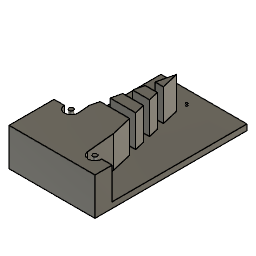
finger_v4_cast_p1 (Autodesk Fusion 360 design; units mm, degrees)
Autodesk Fusion 360 part; units mm, degrees
note: some values were not read from the file. Set by a fixed rule: which sketch regions a step uses.
sketch "Sketch1" plane through (0, 0, 0) normal (0, 0, 1) x (1, 0, 0)
  circle A0 centre (11, 11) radius 1.925
  circle A1 centre (11, 11) radius 3.8
  line L0 (11, 11) -> (56.3, 11) construction
  circle A2 centre (56.3, 11) radius 1.925
  circle A3 centre (56.3, 11) radius 3.8
  line L1 (11, 11) -> (11, 61.7133) construction
  line L2 (11, 11) -> (-8.4114, 83.4444) construction
  line L3 (-8.4114, 83.4444) -> (56.3, 11) construction
  line L4 (11, 11) -> (7.556, 12.6059) construction
  line L5 (11, 11) -> (13.1796, 14.1128) construction
  line L6 (10.0165, 14.6705) -> (8.9812, 18.5342) construction
  line L7 (5.9073, 19.5741) -> (5.1309, 22.4719)
  line L8 (6.3316, 20.3089) -> (5.8657, 22.0476)
  line L9 (5.8657, 22.0476) -> (8.1839, 22.6688)
  line L10 (5.1309, 22.4719) -> (7.4491, 23.093)
  line L11 (8.1839, 22.6688) -> (7.4075, 25.5665)
  line L12 (7.4491, 23.093) -> (6.9832, 24.8317)
  line L13 (6.9832, 24.8317) -> (4.665, 24.2105)
  line L14 (7.4075, 25.5665) -> (5.0893, 24.9454)
  line L15 (4.665, 24.2105) -> (3.8885, 27.1083)
  line L16 (5.0893, 24.9454) -> (4.6234, 26.684)
  line L17 (3.8885, 27.1083) -> (6.2068, 27.7295)
  line L18 (4.6234, 26.684) -> (6.9416, 27.3052)
  line L19 (6.2068, 27.7295) -> (5.7409, 29.4681)
  line L20 (6.9416, 27.3052) -> (6.1652, 30.203)
  line L21 (5.7409, 29.4681) -> (3.4227, 28.847)
  line L22 (6.1652, 30.203) -> (3.8469, 29.5818)
  line L23 (3.4227, 28.847) -> (2.6462, 31.7447)
  line L24 (3.8469, 29.5818) -> (3.3811, 31.3205)
  line L25 (2.6462, 31.7447) -> (4.9644, 32.3659)
  line L26 (3.3811, 31.3205) -> (5.6993, 31.9416)
  line L27 (4.9644, 32.3659) -> (4.4986, 34.1046)
  line L28 (5.6993, 31.9416) -> (4.9228, 34.8394)
  line L29 (4.4986, 34.1046) -> (2.1803, 33.4834)
  line L30 (4.9228, 34.8394) -> (2.6046, 34.2183)
  line L31 (2.1803, 33.4834) -> (1.4039, 36.3812)
  line L32 (2.6046, 34.2183) -> (2.1387, 35.9569)
  line L33 (1.4039, 36.3812) -> (3.7221, 37.0024)
  line L34 (2.1387, 35.9569) -> (4.457, 36.5781)
  line L35 (3.7221, 37.0024) -> (3.2562, 38.741)
  line L36 (4.457, 36.5781) -> (3.6805, 39.4759)
  line L37 (3.2562, 38.741) -> (0.938, 38.1199)
  line L38 (3.6805, 39.4759) -> (1.3623, 38.8547)
  line L39 (0.938, 38.1199) -> (0.1616, 41.0176)
  line L40 (1.3623, 38.8547) -> (0.8964, 40.5934)
  line L41 (0.1616, 41.0176) -> (2.4798, 41.6388)
  line L42 (0.8964, 40.5934) -> (3.2146, 41.2145)
  line L43 (2.4798, 41.6388) -> (2.0139, 43.3775)
  line L44 (3.2146, 41.2145) -> (2.4382, 44.1123)
  line L45 (2.0139, 43.3775) -> (-0.3043, 42.7563)
  line L46 (2.4382, 44.1123) -> (0.1199, 43.4911)
  line L47 (-0.3043, 42.7563) -> (-1.0808, 45.6541)
  line L48 (0.1199, 43.4911) -> (-0.3459, 45.2298)
  line L49 (-1.0808, 45.6541) -> (1.2374, 46.2752)
  line L50 (-0.3459, 45.2298) -> (1.9723, 45.851)
  line L51 (1.2374, 46.2752) -> (0.7716, 48.0139)
  line L52 (1.9723, 45.851) -> (1.1958, 48.7488)
  line L53 (0.7716, 48.0139) -> (-1.5467, 47.3927)
  line L54 (1.1958, 48.7488) -> (-1.1224, 48.1276)
  line L55 (-1.5467, 47.3927) -> (-2.3231, 50.2905)
  line L56 (-1.1224, 48.1276) -> (-1.5883, 49.8663)
  line L57 (-2.3231, 50.2905) -> (-0.0049, 50.9117)
  line L58 (-1.5883, 49.8663) -> (0.73, 50.4874)
  line L59 (-0.0049, 50.9117) -> (-0.4708, 52.6504)
  line L60 (0.73, 50.4874) -> (-0.0465, 53.3852)
  line L61 (-0.4708, 52.6504) -> (-2.789, 52.0292)
  line L62 (-0.0465, 53.3852) -> (-2.3647, 52.764)
  line L63 (-2.789, 52.0292) -> (-3.5654, 54.927)
  line L64 (-2.3647, 52.764) -> (-2.8306, 54.5027)
  line L65 (-3.5654, 54.927) -> (-1.2472, 55.5481)
  line L66 (-2.8306, 54.5027) -> (-0.5124, 55.1239)
  line L67 (-1.2472, 55.5481) -> (-1.7131, 57.2868)
  line L68 (-0.5124, 55.1239) -> (-1.2888, 58.0216)
  line L69 (-1.7131, 57.2868) -> (-4.0313, 56.6656)
  line L70 (-1.2888, 58.0216) -> (-3.607, 57.4005)
  line L71 (-4.0313, 56.6656) -> (-4.8078, 59.5634)
  line L72 (-3.607, 57.4005) -> (-4.0729, 59.1391)
  line L73 (-4.8078, 59.5634) -> (-2.4895, 60.1846)
  line L74 (-4.0729, 59.1391) -> (-1.7547, 59.7603)
  line L75 (-2.4895, 60.1846) -> (-2.9554, 61.9232)
  line L76 (-1.7547, 59.7603) -> (-2.5312, 62.6581)
  line L77 (-2.9554, 61.9232) -> (-5.2736, 61.3021)
  line L78 (-2.5312, 62.6581) -> (-4.8494, 62.0369)
  line L79 (-5.2736, 61.3021) -> (-6.0501, 64.1998)
  line L80 (-4.8494, 62.0369) -> (-5.3153, 63.7756)
  line L81 (-6.0501, 64.1998) -> (-3.7319, 64.821)
  line L82 (-5.3153, 63.7756) -> (-2.997, 64.3968)
  line L83 (-3.7319, 64.821) -> (-4.1978, 66.5597)
  line L84 (-2.997, 64.3968) -> (-3.7735, 67.2945)
  line L85 (-4.1978, 66.5597) -> (-6.516, 65.9385)
  line L86 (-3.7735, 67.2945) -> (-6.0917, 66.6734)
  line L87 (-6.516, 65.9385) -> (-7.2924, 68.8363)
  line L88 (-6.0917, 66.6734) -> (-6.5576, 68.412)
  line L89 (-7.2924, 68.8363) -> (-4.9742, 69.4575)
  line L90 (-6.5576, 68.412) -> (-4.2394, 69.0332)
  line L91 (-4.9742, 69.4575) -> (-5.4401, 71.1961)
  line L92 (-4.2394, 69.0332) -> (-5.0158, 71.931)
  line L93 (-5.4401, 71.1961) -> (-7.7583, 70.575)
  line L94 (-5.0158, 71.931) -> (-7.334, 71.3098)
  line L95 (-7.7583, 70.575) -> (-8.5348, 73.4727)
  line L96 (-7.334, 71.3098) -> (-7.7999, 73.0485)
  line L97 (-8.5348, 73.4727) -> (-6.2165, 74.0939)
  line L98 (-7.7999, 73.0485) -> (-5.4817, 73.6696)
  line L99 (-6.2165, 74.0939) -> (-6.6824, 75.8326)
  line L100 (-5.4817, 73.6696) -> (-6.2582, 76.5674)
  line L101 (-5.4401, 71.1961) -> (-7.7583, 70.575)
  line L102 (-5.0158, 71.931) -> (-7.334, 71.3098)
  line L103 (-7.7583, 70.575) -> (-8.5348, 73.4727)
  line L104 (-7.334, 71.3098) -> (-7.7999, 73.0485)
  line L105 (-8.5348, 73.4727) -> (-6.2165, 74.0939)
  line L106 (-7.7999, 73.0485) -> (-5.4817, 73.6696)
  line L107 (-6.2165, 74.0939) -> (-6.6824, 75.8326)
  line L108 (-5.4817, 73.6696) -> (-6.2582, 76.5674)
  line L109 (-6.6824, 75.8326) -> (-9.0006, 75.2114)
  line L110 (-6.2582, 76.5674) -> (-8.5764, 75.9463)
  line L111 (-8.4114, 83.4444) -> (30.7371, 11) construction
  line L112 (35.3806, 34.8696) -> (37.1705, 36.4685)
  line L113 (34.5334, 34.9174) -> (36.3233, 36.5162)
  line L114 (37.1705, 36.4685) -> (35.1719, 38.7058)
  line L115 (36.3233, 36.5162) -> (35.1242, 37.8587)
  line L116 (35.1719, 38.7058) -> (33.382, 37.107)
  line L117 (35.1242, 37.8587) -> (33.3343, 36.2598)
  line L118 (33.382, 37.107) -> (32.1829, 38.4494)
  line L119 (33.3343, 36.2598) -> (31.3357, 38.4972)
  line L120 (31.3357, 38.4972) -> (33.1256, 40.096)
  line L121 (32.1829, 38.4494) -> (33.9728, 40.0483)
  line L122 (33.9728, 40.0483) -> (31.9743, 42.2856)
  line L123 (33.1256, 40.096) -> (31.9265, 41.4385)
  line L124 (31.9743, 42.2856) -> (30.1844, 40.6868)
  line L125 (31.9265, 41.4385) -> (30.1366, 39.8396)
  line L126 (30.1366, 39.8396) -> (28.1381, 42.077)
  line L127 (30.1844, 40.6868) -> (28.9852, 42.0292)
  line L128 (28.9852, 42.0292) -> (30.7751, 43.6281)
  line L129 (28.1381, 42.077) -> (29.9279, 43.6758)
  line L130 (30.7751, 43.6281) -> (28.7766, 45.8654)
  line L131 (29.9279, 43.6758) -> (28.7288, 45.0182)
  line L132 (28.7766, 45.8654) -> (26.9867, 44.2666)
  line L133 (28.7288, 45.0182) -> (26.9389, 43.4194)
  line L134 (26.9867, 44.2666) -> (25.7876, 45.609)
  line L135 (26.9389, 43.4194) -> (24.9404, 45.6568)
  line L136 (24.9404, 45.6568) -> (26.7303, 47.2556)
  line L137 (25.7876, 45.609) -> (27.5775, 47.2079)
  line L138 (27.5775, 47.2079) -> (25.5789, 49.4452)
  line L139 (26.7303, 47.2556) -> (25.5311, 48.598)
  line L140 (25.5789, 49.4452) -> (23.789, 47.8464)
  line L141 (25.5311, 48.598) -> (23.7413, 46.9992)
  line L142 (23.789, 47.8464) -> (22.5899, 49.1888)
  line L143 (23.7413, 46.9992) -> (21.7427, 49.2366)
  line L144 (22.5899, 49.1888) -> (24.3798, 50.7876)
  line L145 (21.7427, 49.2366) -> (23.5326, 50.8354)
  line L146 (24.3798, 50.7876) -> (22.3812, 53.025)
  line L147 (23.5326, 50.8354) -> (22.3335, 52.1778)
  line L148 (22.3335, 52.1778) -> (20.5436, 50.579)
  line L149 (22.3812, 53.025) -> (20.5913, 51.4262)
  line L150 (20.5913, 51.4262) -> (19.3922, 52.7686)
  line L151 (20.5436, 50.579) -> (18.545, 52.8164)
  line L152 (19.3922, 52.7686) -> (21.1821, 54.3674)
  line L153 (18.545, 52.8164) -> (20.3349, 54.4152)
  line L154 (21.1821, 54.3674) -> (19.1836, 56.6048)
  line L155 (20.3349, 54.4152) -> (19.1358, 55.7576)
  line L156 (19.1836, 56.6048) -> (17.3937, 55.006)
  line L157 (19.1358, 55.7576) -> (17.3459, 54.1588)
  line L158 (17.3937, 55.006) -> (16.1945, 56.3484)
  line L159 (17.3459, 54.1588) -> (15.3474, 56.3962)
  line L160 (15.3474, 56.3962) -> (17.1373, 57.995)
  line L161 (16.1945, 56.3484) -> (17.9844, 57.9472)
  line L162 (17.9844, 57.9472) -> (15.9859, 60.1846)
  line L163 (17.1373, 57.995) -> (15.9381, 59.3374)
  line L164 (15.9381, 59.3374) -> (14.1482, 57.7386)
  line L165 (15.9859, 60.1846) -> (14.196, 58.5858)
  line L166 (14.196, 58.5858) -> (12.9969, 59.9282)
  line L167 (14.1482, 57.7386) -> (12.1497, 59.9759)
  line L168 (12.9969, 59.9282) -> (14.7868, 61.527)
  line L169 (12.1497, 59.9759) -> (13.9396, 61.5748)
  line L170 (14.7868, 61.527) -> (12.7882, 63.7644)
  line L171 (13.9396, 61.5748) -> (12.7405, 62.9172)
  line L172 (12.7882, 63.7644) -> (10.9983, 62.1655)
  line L173 (12.7405, 62.9172) -> (10.9506, 61.3184)
  line L174 (10.9983, 62.1655) -> (9.7992, 63.508)
  line L175 (10.9506, 61.3184) -> (8.952, 63.5557)
  line L176 (9.7992, 63.508) -> (11.5891, 65.1068)
  line L177 (8.952, 63.5557) -> (10.7419, 65.1546)
  line L178 (11.5891, 65.1068) -> (9.5906, 67.3442)
  line L179 (10.7419, 65.1546) -> (9.5428, 66.497)
  line L180 (9.5906, 67.3442) -> (7.8007, 65.7453)
  line L181 (9.5428, 66.497) -> (7.7529, 64.8982)
  line L182 (7.8007, 65.7453) -> (6.6015, 67.0878)
  line L183 (7.7529, 64.8982) -> (5.7544, 67.1355)
  line L184 (5.7544, 67.1355) -> (7.5442, 68.7344)
  line L185 (6.6015, 67.0878) -> (8.3914, 68.6866)
  line L186 (8.3914, 68.6866) -> (6.3929, 70.924)
  line L187 (7.5442, 68.7344) -> (6.3451, 70.0768)
  line L188 (6.3451, 70.0768) -> (4.5552, 68.4779)
  line L189 (6.3929, 70.924) -> (4.603, 69.3251)
  line L190 (4.603, 69.3251) -> (3.4039, 70.6676)
  line L191 (4.5552, 68.4779) -> (2.5567, 70.7153)
  line L192 (3.4039, 70.6676) -> (5.1938, 72.2664)
  line L193 (2.5567, 70.7153) -> (4.3466, 72.3142)
  line L194 (5.1938, 72.2664) -> (3.1952, 74.5038)
  line L195 (4.3466, 72.3142) -> (3.1475, 73.6566)
  line L196 (3.1952, 74.5038) -> (1.4053, 72.9049)
  line L197 (3.1475, 73.6566) -> (1.3576, 72.0577)
  line L198 (1.4053, 72.9049) -> (0.2062, 74.2473)
  line L199 (1.3576, 72.0577) -> (-0.641, 74.2951)
  line L200 (-0.641, 74.2951) -> (1.1489, 75.8939)
  line L201 (0.2062, 74.2473) -> (1.9961, 75.8462)
  line L202 (1.9961, 75.8462) -> (-0.0025, 78.0835)
  line L203 (1.1489, 75.8939) -> (-0.0502, 77.2364)
  line L204 (-0.0025, 78.0835) -> (-1.7923, 76.4847)
  line L205 (-0.0502, 77.2364) -> (-1.8401, 75.6375)
  line L206 (-1.8401, 75.6375) -> (-3.8387, 77.8749)
  line L207 (-1.7923, 76.4847) -> (-2.9915, 77.8271)
  line L208 (-2.9915, 77.8271) -> (-1.2016, 79.426)
  line L209 (-3.8387, 77.8749) -> (-2.0488, 79.4737)
  line L210 (36.5319, 32.68) -> (34.5334, 34.9174)
  line L211 (36.5797, 33.5272) -> (35.3806, 34.8696)
  line L212 (38.3218, 34.2789) -> (36.5319, 32.68)
  line L213 (38.3696, 35.1261) -> (36.5797, 33.5272)
  line L214 (40.3681, 32.8887) -> (38.3696, 35.1261)
  line L215 (39.521, 32.9365) -> (38.3218, 34.2789)
  line L216 (38.5782, 31.2899) -> (40.3681, 32.8887)
  line L217 (37.7311, 31.3376) -> (39.521, 32.9365)
  line L218 (39.7296, 29.1003) -> (37.7311, 31.3376)
  line L219 (39.7774, 29.9474) -> (38.5782, 31.2899)
  line L220 (41.5195, 30.6991) -> (39.7296, 29.1003)
  line L221 (41.5673, 31.5463) -> (39.7774, 29.9474)
  line L222 (43.5658, 29.3089) -> (41.5673, 31.5463)
  line L223 (42.7186, 29.3567) -> (41.5195, 30.6991)
  line L224 (-9.0006, 75.2114) -> (-9.7771, 78.1092)
  line L225 (-8.5764, 75.9463) -> (-9.1975, 78.2645)
  line L226 (-2.0488, 79.4737) -> (-3.6476, 81.2636)
  line L227 (-1.2016, 79.426) -> (-3.2001, 81.6633)
  arc A4 (-3.2001, 81.6633) -> (-9.7771, 78.1092) centre (-6.0657, 79.1036) ccw
  arc A5 (-3.6476, 81.2636) -> (-9.1975, 78.2645) centre (-6.0657, 79.1036) ccw
  line L228 (8.9396, 21.0077) -> (9.5608, 18.6895)
  line L229 (8.4017, 18.3789) -> (7.9358, 20.1176)
  line L230 (5.9073, 19.5741) -> (7.9358, 20.1176)
  line L231 (6.3316, 20.3089) -> (8.9396, 21.0077)
  line L232 (8.4017, 18.3789) -> (9.5608, 18.6895)
  arc A6 (9.5608, 18.6895) -> (13.1796, 14.1128) centre (19.0139, 22.445) ccw
  line L233 (40.705, 27.558) -> (42.3038, 25.7681)
  line L234 (42.3038, 25.7681) -> (43.1988, 26.5675)
  line L235 (43.1988, 26.5675) -> (41.9996, 27.9099)
  line L236 (41.9996, 27.9099) -> (43.5658, 29.3089)
  line L237 (40.705, 27.558) -> (42.7186, 29.3567)
  line L238 (43.1988, 26.5675) -> (58.6993, 13.9468)
  line L239 (42.3038, 25.7681) -> (53.1022, 8.9471)
  line L240 (-9.7771, 78.1092) -> (-12.1919, 77.4621) construction
  line L241 (-3.2001, 81.6633) -> (-1.3357, 83.3288) construction
  line L242 (43.5658, 29.3089) -> (45.4303, 30.9744) construction
  line L243 (5.9073, 19.5741) -> (3.4925, 18.927) construction
  line L244 (3.4925, 18.927) -> (-12.1919, 77.4621)
  line L245 (-1.3357, 83.3288) -> (45.4303, 30.9744)
  arc A7 (-1.3357, 83.3288) -> (-12.1919, 77.4621) centre (-6.0657, 79.1036) ccw
  line L246 (8.9396, 21.0077) -> (10.3885, 21.396) construction
  line L247 (40.705, 27.558) -> (39.5863, 26.5587) construction
  line L248 (10.3885, 21.396) -> (-4.0991, 75.4645)
  line L249 (-4.0991, 75.4645) -> (39.5863, 26.5587)
  circle A8 centre (11, 11) radius 5.5 construction
  line L250 (5.9772, 9.6541) -> (3.4925, 18.927)
  circle A9 centre (11, 11) radius 5.2
  line L251 (10.3885, 21.396) -> (15.3451, 13.8566)
  arc A10 (7.556, 12.6059) -> (8.4017, 18.3789) centre (-1.6628, 16.9047) ccw
  line L252 (45.4303, 30.9744) -> (60.1781, 14.4642)
  line L253 (39.5863, 26.5587) -> (51.9832, 8.1007)
  line L254 (-0.5124, 55.1239) -> (10.9506, 61.3184)
  line L255 (3.2146, 41.2145) -> (20.5436, 50.579)
  line L256 (6.9416, 27.3052) -> (30.1366, 39.8396)
  line L257 (5.3111, 33.3905) -> (25.9397, 44.5381)
  line L258 (1.5841, 47.2999) -> (16.3466, 55.2775)
  line L259 (-2.1429, 61.2092) -> (6.7536, 66.0168)
  line L260 (-8.4114, 83.4444) -> (-9.0809, 84.6834) construction
  line L261 (-9.0809, 84.6834) -> (-12.8843, 91.7215) construction
  line L262 (-12.8843, 91.7215) -> (18.5137, 108.6887)
  line L263 (-12.8843, 91.7215) -> (-39.7732, 77.1909)
  line L264 (-39.7732, 77.1909) -> (15.9015, -25.8352)
  line L265 (18.5137, 108.6887) -> (74.1884, 5.6627)
  line L266 (15.9015, -25.8352) -> (74.1884, 5.6627)
  line L267 (58.7722, 6.4252) -> (62.5755, -0.6129) construction
  line L268 (6.4252, 8.5278) -> (-0.6128, 4.7245)
  line L269 (52.8358, 14.8781) -> (49.4579, 11.8607)
  line L270 (52.8359, 14.8781) -> (56.714, 18.3423)
  arc A11 (51.9832, 8.1007) -> (60.1781, 14.4642) centre (56.3, 11) ccw
  line L271 (55.0864, 16.8884) -> (50.5853, 12.8678)
  circle A12 centre (56.3, 11) radius 1.725
  circle A13 centre (11, 11) radius 1.725
  line L272 (60.8748, 13.4722) -> (67.9129, 17.2755)
  line L273 (-7.8924, 82.484) -> (-7.6072, 81.9561) construction
  circle A14 centre (-7.7498, 82.22) radius 0.8
  point P0 (5.9772, 9.6541)
  point P1 (58.7722, 6.4252)
  point P2 (6.4252, 8.5278)
  point P3 (60.8748, 13.4722)
  dimension "d1" = 3.85
  dimension "d2" = 7.6
  dimension "d3" = 45.3
  dimension "d4" = 3.85
  dimension "d5" = 7.6
  dimension "d6" = 75
  dimension "d7" = 15
  dimension "d8" = 50
  dimension "d9" = 50
  dimension "d10" = 4
  dimension "d23" = 13.386
  dimension "d56" = 24.5
  dimension "d57" = 0
  dimension "d65" = 2.5
  dimension "d66" = 2.5
  dimension "d67" = 2.5
  dimension "d68" = 2.5
  dimension "d69" = 1.5
  dimension "d70" = 1.5
  dimension "d71" = 11
  dimension "d73" = 8
  dimension "d79" = 8
  dimension "d80" = 8
  dimension "d81" = 5.2
  dimension "d82" = 8
  dimension "d83" = 3.45
  dimension "d84" = 3.45
  dimension "d91" = 1.6
  constraint concentric A0 A1
  constraint coincident A0.centre A1.centre
  constraint horizontal L0
  constraint coincident L0.end A2.centre
  constraint concentric A2 A3
  constraint perpendicular L0 L1
  constraint coincident L1.end L3
  constraint coincident A1 L4.end
  constraint coincident A1 L5.end
  constraint coincident A1 L6.start
  constraint coincident L2 L6.start
  constraint parallel L2 L6
  constraint perpendicular L8 L9
  constraint perpendicular L2 L10
  constraint perpendicular L9 L11
  constraint perpendicular L10 L12
  constraint perpendicular L13 L15
  constraint perpendicular L14 L16
  constraint perpendicular L16 L18
  constraint perpendicular L18 L20
  constraint perpendicular L17 L19
  constraint perpendicular L21 L23
  constraint perpendicular L22 L24
  constraint perpendicular L24 L26
  constraint perpendicular L26 L28
  constraint perpendicular L25 L27
  constraint perpendicular L29 L31
  constraint perpendicular L30 L32
  constraint perpendicular L32 L34
  constraint perpendicular L34 L36
  constraint perpendicular L33 L35
  constraint perpendicular L37 L39
  constraint perpendicular L38 L40
  constraint perpendicular L40 L42
  constraint perpendicular L42 L44
  constraint perpendicular L41 L43
  constraint perpendicular L45 L47
  constraint perpendicular L46 L48
  constraint perpendicular L48 L50
  constraint perpendicular L50 L52
  constraint perpendicular L49 L51
  constraint perpendicular L53 L55
  constraint perpendicular L54 L56
  constraint perpendicular L56 L58
  constraint perpendicular L58 L60
  constraint perpendicular L57 L59
  constraint perpendicular L61 L63
  constraint perpendicular L62 L64
  constraint perpendicular L64 L66
  constraint perpendicular L66 L68
  constraint perpendicular L65 L67
  constraint perpendicular L69 L71
  constraint perpendicular L70 L72
  constraint perpendicular L72 L74
  constraint perpendicular L74 L76
  constraint perpendicular L73 L75
  constraint perpendicular L77 L79
  constraint perpendicular L78 L80
  constraint perpendicular L80 L82
  constraint perpendicular L82 L84
  constraint perpendicular L81 L83
  constraint perpendicular L85 L87
  constraint perpendicular L86 L88
  constraint perpendicular L88 L90
  constraint perpendicular L90 L92
  constraint perpendicular L89 L91
  constraint perpendicular L93 L95
  constraint perpendicular L94 L96
  constraint perpendicular L96 L98
  constraint perpendicular L98 L100
  constraint perpendicular L97 L99
  constraint perpendicular L101 L103
  constraint perpendicular L102 L104
  constraint perpendicular L104 L106
  constraint perpendicular L106 L108
  constraint perpendicular L105 L107
  constraint coincident L0 L111.end
  constraint symmetric L7.start L111 L112.end
  constraint symmetric L7.end L111 L114.end
  constraint symmetric L8.start L111 L113.end
  constraint symmetric L8.end L111 L115.end
  constraint symmetric L9.end L111 L117.end
  constraint symmetric L10.end L111 L116.end
  constraint symmetric L11.end L111 L119.end
  constraint symmetric L12.end L111 L118.end
  constraint symmetric L15.end L111 L122.end
  constraint symmetric L19.end L111 L127.end
  constraint symmetric L16.end L111 L123.end
  constraint symmetric L18.end L111 L125.end
  constraint symmetric L20.end L111 L126.end
  constraint symmetric L17.end L111 L124.end
  constraint symmetric L13.end L111 L121.end
  constraint symmetric L14.end L111 L120.end
  constraint symmetric L23.end L111 L130.end
  constraint symmetric L27.end L111 L134.end
  constraint symmetric L24.end L111 L131.end
  constraint symmetric L28.end L111 L135.end
  constraint symmetric L36.end L111 L143.end
  constraint symmetric L33.end L111 L140.end
  constraint symmetric L26.end L111 L133.end
  constraint symmetric L34.end L111 L141.end
  constraint symmetric L31.end L111 L138.end
  constraint symmetric L25.end L111 L132.end
  constraint symmetric L21.end L111 L128.end
  constraint symmetric L32.end L111 L139.end
  constraint symmetric L35.end L111 L142.end
  constraint symmetric L29.end L111 L137.end
  constraint symmetric L30.end L111 L136.end
  constraint symmetric L22.end L111 L129.end
  constraint symmetric L39.end L111 L146.end
  constraint symmetric L43.end L111 L150.end
  constraint symmetric L40.end L111 L147.end
  constraint symmetric L44.end L111 L151.end
  constraint symmetric L52.end L111 L159.end
  constraint symmetric L49.end L111 L156.end
  constraint symmetric L42.end L111 L148.end
  constraint symmetric L50.end L111 L157.end
  constraint symmetric L47.end L111 L154.end
  constraint symmetric L41.end L111 L149.end
  constraint symmetric L37.end L111 L144.end
  constraint symmetric L48.end L111 L155.end
  constraint symmetric L51.end L111 L158.end
  constraint symmetric L45.end L111 L152.end
  constraint symmetric L46.end L111 L153.end
  constraint symmetric L38.end L111 L145.end
  constraint symmetric L55.end L111 L162.end
  constraint symmetric L59.end L111 L166.end
  constraint symmetric L56.end L111 L163.end
  constraint symmetric L60.end L111 L167.end
  constraint symmetric L68.end L111 L175.end
  constraint symmetric L65.end L111 L172.end
  constraint symmetric L58.end L111 L164.end
  constraint symmetric L66.end L111 L173.end
  constraint symmetric L63.end L111 L170.end
  constraint symmetric L57.end L111 L165.end
  constraint symmetric L53.end L111 L161.end
  constraint symmetric L64.end L111 L171.end
  constraint symmetric L67.end L111 L174.end
  constraint symmetric L61.end L111 L168.end
  constraint symmetric L62.end L111 L169.end
  constraint symmetric L54.end L111 L160.end
  constraint symmetric L71.end L111 L178.end
  constraint symmetric L75.end L111 L182.end
  constraint symmetric L72.end L111 L179.end
  constraint symmetric L76.end L111 L183.end
  constraint symmetric L84.end L111 L191.end
  constraint symmetric L81.end L111 L189.end
  constraint symmetric L74.end L111 L181.end
  constraint symmetric L82.end L111 L188.end
  constraint symmetric L79.end L111 L186.end
  constraint symmetric L73.end L111 L180.end
  constraint symmetric L69.end L111 L176.end
  constraint symmetric L80.end L111 L187.end
  constraint symmetric L83.end L111 L190.end
  constraint symmetric L77.end L111 L185.end
  constraint symmetric L78.end L111 L184.end
  constraint symmetric L70.end L111 L177.end
  constraint symmetric L87.end L111 L194.end
  constraint symmetric L91.end L111 L198.end
  constraint symmetric L88.end L111 L195.end
  constraint symmetric L92.end L111 L199.end
  constraint symmetric L97.end L111 L204.end
  constraint symmetric L90.end L111 L197.end
  constraint symmetric L95.end L111 L202.end
  constraint symmetric L89.end L111 L196.end
  constraint symmetric L85.end L111 L192.end
  constraint symmetric L93.end L111 L201.end
  constraint symmetric L94.end L111 L200.end
  constraint symmetric L86.end L111 L193.end
  constraint symmetric L98.end L111 L205.end
  constraint symmetric L100.end L111 L206.end
  constraint symmetric L96.end L111 L203.end
  constraint symmetric L99.end L111 L207.end
  constraint symmetric L110.end L111 L209.end
  constraint symmetric L109.end L111 L208.end
  constraint perpendicular L109 L224
  constraint perpendicular L110 L225
  constraint perpendicular L209 L226
  constraint perpendicular L208 L227
  constraint tangent L227 A4
  constraint tangent L224 A4
  constraint tangent L226 A5
  constraint tangent L225 A5
  constraint perpendicular L229 L230
  constraint perpendicular L228 L231
  constraint perpendicular L228 L232
  constraint tangent A1 A6
  constraint perpendicular L222 L236
  constraint perpendicular L223 L237
  constraint coincident A3 L238.end
  constraint tangent A3 L238
  constraint coincident A3 L239.end
  constraint tangent A3 L239
  constraint perpendicular L224 L240
  constraint perpendicular L227 L241
  constraint perpendicular L222 L242
  constraint perpendicular L7 L243
  constraint perpendicular L240 L244
  constraint perpendicular L242 L245
  constraint tangent L245 A7
  constraint perpendicular L228 L246
  constraint perpendicular L233 L247
  constraint coincident L111 L248.end
  constraint perpendicular L102 L248
  constraint coincident P0 L250.start
  constraint perpendicular L243 L250
  constraint coincident P0 A9
  constraint tangent L250 A9
  constraint coincident A9 L251.end
  constraint tangent A9 L251
  constraint tangent A1 A10
  constraint perpendicular L242 L252
  constraint midpoint L28 L257.start
  constraint midpoint L135 L257.end
  constraint midpoint L52 L258.start
  constraint midpoint L159 L258.end
  constraint midpoint L76 L259.start
  constraint midpoint L183 L259.end
  constraint midpoint A7 L260.end
  constraint parallel L260 L261
  constraint perpendicular L261 L262
  constraint perpendicular L261 L263
  constraint perpendicular L263 L264
  constraint perpendicular L262 L265
  constraint perpendicular L265 L266
  constraint coincident P1 L267.start
  constraint coincident L266 L267.end
  constraint perpendicular L266 L267
  constraint coincident A9 P2
  constraint coincident P2 L268.start
  constraint coincident L264 L268.end
  constraint perpendicular L264 L268
  constraint coincident L3 L269.start
  constraint coincident L253 L269.end
  constraint perpendicular L3 L269
  constraint coincident L252 L270.end
  constraint coincident A11 P3
  constraint coincident L270 L271.start
  constraint coincident L238 L271.start
  constraint coincident L239 L271.end
  constraint coincident L269 L271.end
  constraint concentric A2 A12
  constraint concentric A0 A13
  constraint coincident P3 L272.start
  constraint coincident L265 L272.end
  constraint perpendicular L265 L272
  constraint midpoint A4 L273.start
  constraint midpoint A5 L273.end
  constraint parallel L111 L273
  constraint midpoint L273 A14.centre
  measures "d1" diameter of A0
  measures "d2" diameter of A1
  measures "d3" distance of A0.centre L0.end
  measures "d4" diameter of A2
  measures "d5" diameter of A3
  measures "d6" distance of A0.centre L2.end
  measures "d7" angle of L1 L2
  measures "d8" angle of L2 L4
  measures "d9" angle of L2 L5
  measures "d10" distance of L6.start L6.end
  measures "d23" angle of L3 L111
  measures "d65" distance of L222.start L242.end
  measures "d66" distance of L7.start L243.end
  measures "d67" distance of L224.end L240.end
  measures "d68" distance of L227.end L241.end
  measures "d69" distance of L228.start L246.end
  measures "d70" distance of L233.start L247.end
  measures "d71" diameter of A8
  measures "d73" distance of L260.end L261.end
  measures "d79" distance of P1 L267.end
  measures "d80" distance of P2 L268.end
  measures "d81" distance of L0.end L270.start
  measures "d82" distance of L265 P3
  measures "d83" diameter of A12
  measures "d84" diameter of A13
  measures "d91" diameter of A14
extrude "Extrude6" add sketch "Sketch1" along normal blind 4.5 contours A0 | A1 | A1 A6 A9 A10 | A1 A6 A9 A10 | L232 A6 A9 A10 | L8 L9 L11 L14 L16 L18 L228 L231 A6 L248 A9 L251 L256 | L7 L10 L12 L13 L15 L17 L19 L21 L23 L25 L27 L29 L31 L33 L35 L37 L39 L41 L43 L45 L47 L49 L51 L53 L55 L57 L59 L61 L63 L65 L67 L69 L71 L73 L75 L77 L79 L81 L83 L85 L87 L89 L91 L93 L95 L97 L99 L101 L103 L105 L107 L109 L112 L114 L116 L118 L121 L122 L124 L127 L128 L130 L132 L134 L137 L138 L140 L142 L144 L146 L149 L150 L152 L154 L156 L158 L161 L162 L165 L166 L168 L170 L172 L174 L176 L178 L180 L182 L185 L186 L189 L190 L192 L194 L196 L198 L201 L202 L204 L207 L208 L211 L213 L214 L216 L219 L221 L222 L224 L227 A4 L229 L230 L235 L236 L238 L244 L245 A7 L250 A9 A10 L252 L270 A14 | L7 L8 L9 L10 L11 L12 L13 L14 L15 L16 L17 L18 L19 L20 L21 L22 L23 L24 L25 L26 L27 L28 L29 L30 L31 L32 L33 L34 L35 L36 L37 L38 L39 L40 L41 L42 L43 L44 L45 L46 L47 L48 L49 L50 L51 L52 L53 L54 L55 L56 L57 L58 L59 L60 L61 L62 L63 L64 L65 L66 L67 L68 L69 L70 L71 L72 L73 L74 L75 L76 L77 L78 L79 L80 L81 L82 L83 L84 L85 L86 L87 L88 L89 L90 L91 L92 L93 L94 L95 L96 L97 L98 L99 L100 L101 L102 L103 L104 L105 L106 L107 L108 L109 L110 L224 L225 A4 A5 L228 L229 L230 L231 L232 A14 | L244 L245 A7 L250 A9 L252 L262 L263 L264 L265 L268 A11 L272 | L20 L22 L24 L26 L28 L248 L256 L257 | L248 L249 L256 L257 | L28 L30 L32 L34 L36 L38 L40 L42 L248 L255 L257 | L113 L115 L117 L119 L120 L123 L125 L210 L212 L215 L217 L218 L220 L223 L233 L237 L239 L249 L253 L256 L269 | L126 L129 L131 L133 L135 L249 L256 L257 | L44 L46 L48 L50 L52 L248 L255 L258 | L248 L249 L255 L258 | L135 L136 L139 L141 L143 L145 L147 L148 L249 L255 L257 | L112 L113 L114 L115 L116 L117 L118 L119 L120 L121 L122 L123 L124 L125 L126 L127 L128 L129 L130 L131 L132 L133 L134 L135 L136 L137 L138 L139 L140 L141 L142 L143 L144 L145 L146 L147 L148 L149 L150 L151 L152 L153 L154 L155 L156 L157 L158 L159 L160 L161 L162 L163 L164 L165 L166 L167 L168 L169 L170 L171 L172 L173 L174 L175 L176 L177 L178 L179 L180 L181 L182 L183 L184 L185 L186 L187 L188 L189 L190 L191 L192 L193 L194 L195 L196 L197 L198 L199 L200 L201 L202 L203 L204 L205 L206 L207 L208 L209 L210 L211 L212 L213 L214 L215 L216 L217 L218 L219 L220 L221 L222 L223 L226 L227 A4 A5 L233 L234 L235 L236 L237 A14 | L52 L54 L56 L58 L60 L62 L64 L66 L248 L254 L258 | L151 L153 L155 L157 L159 L249 L255 L258 | A3 L238 L239 L252 L253 L269 L270 A11 | L68 L70 L72 L74 L76 L248 L254 L259 | L248 L249 L254 L259 | L159 L160 L163 L164 L167 L169 L171 L173 L249 L254 L258 | A3 L238 L239 L269 L270 L271 | L234 L238 L239 L269 L270 L271 | L76 L78 L80 L82 L84 L86 L88 L90 L92 L94 L96 L98 L100 L102 L104 L106 L108 L110 L183 L184 L187 L188 L191 L193 L195 L197 L199 L200 L203 L205 L206 L209 L225 L226 A5 L248 L249 L259 A14 | L175 L177 L179 L181 L183 L249 L254 L259 | A3 | A4 A5 A14 | A5 A14 | A4 A14 | A2
extrude "Extrude7" add sketch "Sketch1" along normal blind 29 contours L248 L249 A9 L251 L253 L256 L264 L265 L266 L268 A11 L272 | L248 L249 L255 L257 | L248 L249 L254 L258 | L248 L249 L259 | A12 | A13
extrude "Extrude8" add sketch "Sketch1" along normal blind 5.75 contours A0 | A1 | A3 | A2
extrude "Extrude9" add sketch "Sketch1" along normal blind 5.75 contours A4 A5 A14 | A5 A14 | A4 A14
move_body "Align3" bodies 1 to x (0.879761, -0.475417, 0) y (0.475417, 0.879761, 0) z (0, 0, 1) at (14.1945, 30.2886, 0)
